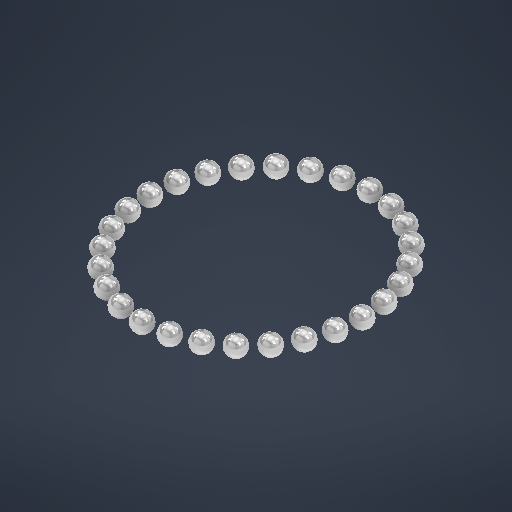
# Autodesk Inventor part: 2.5mm_BALL_BEARINGS
Saved by Autodesk Inventor 2026.2 (Build 302298010, 298A)
## iProperties
Created: 2026-03-05
Part Number: 2.5mm_BALL_BEARINGS
Material: Steel, O1, HT 58-60 Rc
Document SubType Name: Modeling
Designer: 4aida
Density: 7.86 g/cm^3
Appearance: Chrome - Polished
Author: 4aida
Autodesk Inventor part; units mm, degrees
ref_plane "YZ Plane" through (0, 0, 0) normal (1, 0, 0) x (0, 1, 0)
ref_plane "XZ Plane" through (0, 0, 0) normal (0, 1, 0) x (-1, 0, 0)
ref_plane "XY Plane" through (0, 0, 0) normal (0, 0, 1) x (1, 0, 0)
sketch "Sketch1" plane through (0, 0, 0) normal (1, 0, 0) x (0, 1, 0)
  line L0 (-1.25, 14.95) -> (1.25, 14.95)
  arc A0 (1.25, 14.95) -> (-1.25, 14.95) centre (0, 14.95) ccw
  point P0 (0, 0)
  point P1 (0, 0)
  point P2 (0, 16.2)
  dimension "d5" = 1.25
  dimension "d14" = 16.2
  constraints: 3 point on circle, 2 end point, 1 centre point, 1 horizontal, 1 line through centre, 1 vertical alignment
  measures "d5" radius of A0
  measures "d14" distance of point (0, 0) point (0, 16.2)
revolve "Revolution1" add sketch "Sketch1" angle 360 about axis through (0, -1.25, 14.95) along (0, 1, 0)
pattern_sketch "Sketch Driven Pattern2" of "Revolution1" from (0, 0, 14.95) copies at (-3.2117, 0, 14.5484) at (-6.2289, 0, 13.3769) at (-8.8843, 0, 11.5261) at (-11.0519, 0, 9.1224) at (-12.648, 0, 6.3066) at (-13.6226, 0, 3.2201) at (-13.95, 0, 0) at (-13.6226, 0, -3.2201) at (-12.648, 0, -6.3066) at (-11.0519, 0, -9.1224) at (-8.8843, 0, -11.526) at (-6.229, 0, -13.3768) at (-3.2118, 0, -14.5484) at (3.2118, 0, -14.5484) at (6.229, 0, -13.3768) at (8.8843, 0, -11.526) at (11.0519, 0, -9.1224) at (12.648, 0, -6.3066) at (13.6226, 0, -3.2201) at (13.95, 0, 0) at (13.6226, 0, 3.2201) at (12.648, 0, 6.3066) at (11.0519, 0, 9.1224) at (8.8843, 0, 11.5261) at (6.2289, 0, 13.3769) at (3.2117, 0, 14.5484) at (0.0001, 0, -14.95)
sketch "Sketch3" plane through (0, 0, 0) normal (0, 1, 0) x (-1, 0, 0)
  ellipse E0 centre (0, 0) end of major axis (0, 14.95) minor radius 13.95 construction
  circle A0 centre (0, 14.95) radius 1.25 construction
  line L0 (0, 14.95) -> (0, 0) construction
  line L1 (0, 0) -> (13.95, 0) construction
  circle A1 centre (0.0001, -14.95) radius 1.25 construction
  circle A2 centre (0, 14.95) radius 1.25 construction
  line L2 (0, 0) -> (-13.95, 0) construction
  point P0 (3.2117, 14.5484)
  point P1 (6.2289, 13.3769)
  point P2 (8.8843, 11.5261)
  point P3 (11.0519, 9.1224)
  point P4 (12.648, 6.3066)
  point P5 (13.6226, 3.2201)
  point P6 (3.2118, -14.5484)
  point P7 (6.229, -13.3768)
  point P8 (8.8843, -11.526)
  point P9 (11.0519, -9.1224)
  point P10 (12.648, -6.3066)
  point P11 (13.6226, -3.2201)
  point P12 (-3.2117, 14.5484)
  point P13 (-6.2289, 13.3769)
  point P14 (-8.8843, 11.5261)
  point P15 (-11.0519, 9.1224)
  point P16 (-12.648, 6.3066)
  point P17 (-13.6226, 3.2201)
  point P18 (-0.0001, -14.95)
  point P19 (-13.6226, -3.2201)
  point P20 (-12.648, -6.3066)
  point P21 (-11.0519, -9.1224)
  point P22 (-8.8843, -11.526)
  point P23 (-6.229, -13.3768)
  point P24 (-3.2118, -14.5484)
  point P25 (-0.0001, -14.95)
  dimension "d15" = 13.95
  dimension "d7" = 3.2367
  dimension "d8" = 3.2367
  dimension "d9" = 3.2367
  dimension "d10" = 3.2367
  dimension "d11" = 3.2367
  dimension "d12" = 3.2367
  dimension "d13" = 3.2367
  constraints: 21 symmetric about line, 6 end point, 3 coincident, 2 centre point, 1 vertical, 12 other
  measures "d7" distance of L0.start point (3.212, 14.548)
  measures "d8" distance of point (6.229, 13.377) point (3.212, 14.548)
  measures "d9" distance of point (8.884, 11.526) point (6.229, 13.377)
  measures "d10" distance of point (8.884, 11.526) point (11.052, 9.122)
  measures "d11" distance of point (11.052, 9.122) point (12.648, 6.307)
  measures "d12" distance of point (13.623, 3.22) point (12.648, 6.307)
  measures "d13" distance of L1.end point (13.623, 3.22)
equation "\"d8\" = d7"
equation "\"d9\" = d8"
equation "\"d10\" = d9"
equation "\"d11\" = d10"
equation "\"d12\" = d11"
equation "\"d13\" = d12"
body "Solid1"
